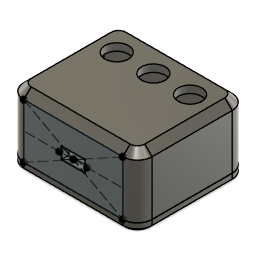
Button game box v5 (Autodesk Fusion 360 design; units mm, degrees)
Autodesk Fusion 360 part; units mm, degrees
sketch "Sketch2" plane through (0, 0, 0) normal (0, 1, 0) x (1, 0, 0)
  line L0 (-40.8037, -70.8274) -> (-40.8037, -26.2061)
  line L1 (-40.3037, -48.0998) -> (36.1963, -48.0998) construction
  line L2 (36.1963, -48.0998) -> (36.1963, -70.0998) construction
  line L3 (36.1963, -70.0998) -> (-40.3037, -70.0998) construction
  line L4 (-40.3037, -70.0998) -> (-40.3037, -48.0998) construction
  line L5 (-37.3037, -23.6203) -> (32.6963, -23.6203) construction
  line L6 (32.6963, -23.6203) -> (32.6963, -73.6203) construction
  line L7 (32.6963, -73.6203) -> (-37.3037, -73.6203) construction
  line L8 (-37.3037, -73.6203) -> (-37.3037, -23.6203) construction
  line L9 (36.1963, -48.0998) -> (-40.3037, -70.0998) construction
  line L10 (36.1963, -70.0998) -> (-40.3037, -48.0998) construction
  circle A0 centre (-2.0537, -59.0998) radius 2
  line L11 (30.6963, -23.6203) -> (30.6963, -73.6203) construction
  circle A1 centre (27.6642, -69.1203) radius 1.25
  line L12 (32.6963, -48.6203) -> (-37.3037, -48.6203) construction
  circle A2 centre (27.6642, -28.1203) radius 1.25
  line L13 (31.6963, -85.8274) -> (-35.8037, -85.8274)
  line L14 (-45.8037, -75.8274) -> (-45.8037, -21.2061)
  line L15 (-35.8037, -11.2061) -> (31.6963, -11.2061)
  line L16 (41.6963, -21.2061) -> (41.6963, -75.8274)
  arc A3 (-35.8037, -11.2061) -> (-45.8037, -21.2061) centre (-35.8037, -21.2061) ccw
  arc A4 (-45.8037, -75.8274) -> (-35.8037, -85.8274) centre (-35.8037, -75.8274) ccw
  arc A5 (31.6963, -85.8274) -> (41.6963, -75.8274) centre (31.6963, -75.8274) ccw
  arc A6 (41.6963, -21.2061) -> (31.6963, -11.2061) centre (31.6963, -21.2061) ccw
  line L17 (25.6941, -69.8252) -> (38.7674, -82.8985) construction
  line L18 (-35.8037, -75.8274) -> (-42.8747, -82.8985) construction
  line L19 (-35.8037, -75.8274) -> (-29.9973, -70.021) construction
  circle A7 centre (-39.3392, -79.3629) radius 2
  line L20 (25.6941, -69.8252) -> (15.45, -59.5811) construction
  circle A8 centre (35.2319, -79.3629) radius 2
  line L21 (38.7674, -14.135) -> (39.7345, -13.168) construction
  line L22 (39.7345, -13.168) -> (31.6963, -21.2061) construction
  circle A9 centre (35.2319, -17.6705) radius 2
  line L23 (-42.8747, -14.135) -> (-49.8297, -7.18) construction
  line L24 (-49.8297, -7.18) -> (-35.8037, -21.2061) construction
  circle A10 centre (-39.3392, -17.6705) radius 2
  line L25 (26.6963, -80.8274) -> (36.6963, -70.8274)
  line L26 (36.6963, -26.2061) -> (36.6963, -70.8274)
  line L27 (-40.8037, -70.8274) -> (-30.8037, -80.8274)
  line L28 (-40.8037, -26.2061) -> (-30.8037, -16.2061)
  line L29 (26.6963, -16.2061) -> (36.6963, -26.2061)
  line L30 (-30.8037, -16.2061) -> (26.6963, -16.2061)
  line L31 (26.6963, -80.8274) -> (-30.8037, -80.8274)
  circle A11 centre (-39.3392, -79.3629) radius 1.6
  circle A12 centre (-39.3392, -17.6705) radius 1.6
  circle A13 centre (35.2319, -17.6705) radius 1.6
  circle A14 centre (35.2319, -79.3629) radius 1.6
  dimension "d25" = 76.5
  dimension "d26" = 22
  dimension "d27" = 50
  dimension "d28" = 70
  dimension "d29" = 0.5
  dimension "d30" = 0.5
  dimension "d32" = 4
  dimension "d33" = 2.5
  dimension "d34" = 41
  dimension "d35" = 6
  dimension "d36" = 4
  dimension "d40" = 10
  dimension "d50" = 4
  dimension "d51" = 5
  dimension "d53" = 4
  dimension "d54" = 5
  dimension "d55" = 4
  dimension "d56" = 4
  dimension "d57" = 5
  dimension "d58" = 5
  dimension "d59" = 45
  dimension "d60" = 5
  dimension "d65" = 45
  dimension "d66" = 5
  dimension "d69" = 5
  dimension "d70" = 5
  dimension "d71" = 5
  dimension "d72" = 0.5
  dimension "d73" = 135
  dimension "d74" = 135
  dimension "d78" = 1
  dimension "d91" = 15.7276
  dimension "d105" = 3.2
  dimension "d106" = 3.2
  dimension "d107" = 3.2
  dimension "d108" = 3.2
  constraint vertical L26
  constraint horizontal L31
  constraint vertical L0
  constraint horizontal L1
  constraint vertical L2
  constraint horizontal L3
  constraint vertical L4
  constraint horizontal L5
  constraint vertical L6
  constraint horizontal L7
  constraint vertical L8
  constraint midpoint L9 A0.centre
  constraint coincident L5 L11.start
  constraint coincident L7 L11.end
  constraint perpendicular L7 L11
  constraint midpoint L6 L12.start
  constraint midpoint L8 L12.end
  constraint symmetric A1 L12 A2
  constraint tangent L15 A3
  constraint tangent L14 A3
  constraint tangent L14 A4
  constraint tangent L13 A4
  constraint equal A3 A4
  constraint tangent L13 A5
  constraint tangent L16 A5
  constraint equal A3 A5
  constraint tangent L16 A6
  constraint tangent L15 A6
  constraint equal A3 A6
  constraint midpoint A5 L17.end
  constraint midpoint A4 L18.end
  constraint parallel L18 L19
  constraint coincident L19 A7.centre
  constraint collinear L17 L20
  constraint coincident L20 A8.centre
  constraint midpoint A6 L21.start
  constraint coincident A6.centre L22.end
  constraint coincident L22 A9.centre
  constraint midpoint A3 L23.start
  constraint coincident A3.centre L24.end
  constraint coincident L23 A10.centre
  constraint horizontal L15
  constraint horizontal L30
  constraint midpoint A4.centre L27
  constraint perpendicular L17 L25
  constraint perpendicular L22 L29
  constraint perpendicular L24 L28
  constraint concentric A7 A11
  constraint concentric A10 A12
  constraint concentric A9 A13
  constraint concentric A8 A14
  measures "d25" distance of L2 L4
  measures "d26" distance of L1 L3
  measures "d27" distance of L5 L7
  measures "d28" distance of L6 L8
  measures "d29" distance of L2 L26
  measures "d30" distance of L0 L4
  measures "d32" diameter of A0
  measures "d33" diameter of A1
  measures "d34" distance of A1.centre A2.centre
  measures "d35" distance of L11 L26
  measures "d36" distance of L6 L26
  measures "d40" radius of A3
  measures "d50" diameter of A7
  measures "d51" distance of L18.end A7.centre
  measures "d53" diameter of A8
  measures "d54" distance of L17.end A8.centre
  measures "d55" diameter of A9
  measures "d56" diameter of A10
  measures "d57" distance of L23.start A10.centre
  measures "d58" distance of L21.start A9.centre
  measures "d59" angle of L25 L31
  measures "d60" distance of A8.centre L25
  measures "d65" angle of L27 L31
  measures "d66" distance of A7.centre L27
  measures "d69" distance of A10.centre L28
  measures "d70" distance of A9.centre L29
  measures "d71" distance of L15 L30
  measures "d72" distance of L7.end L27
  measures "d73" angle of L28 L30
  measures "d74" angle of L29 L30
  measures "d78" distance of L5.end L29
  measures "d91" distance of L3 L13
  measures "d105" diameter of A11
  measures "d106" diameter of A12
  measures "d107" diameter of A13
  measures "d108" diameter of A14
extrude "Extrude4" add sketch "Sketch2" against normal blind 5 contours L0 L25 L26 L27 L28 L29 L30 L31 | A0 | A1 | A2 | L13 L14 L15 L16 A3 A4 A5 A6 | A7 | A8 | A9 | A10 | A11 | A12 | A13 | A14 makes body 1
extrude "Extrude5" add sketch "Sketch2" against normal blind 37 from surface at -5 contours L13 L14 L15 L16 A3 A4 A5 A6 | A7 | A8 | A9 | A10 | A11 | A12 | A13 | A14 bodies 1
sketch "Sketch1" plane through (0, 0, 0) normal (0, 1, 0) x (1, 0, 0)
  arc A0 (31.6963, -85.8274) -> (41.6963, -75.8274) centre (31.6963, -75.8274) ccw
  line L0 (41.6963, -75.8274) -> (41.6963, -21.2061)
  arc A1 (41.6963, -21.2061) -> (31.6963, -11.2061) centre (31.6963, -21.2061) ccw
  line L1 (31.6963, -11.2061) -> (-35.8037, -11.2061)
  arc A2 (-35.8037, -11.2061) -> (-45.8037, -21.2061) centre (-35.8037, -21.2061) ccw
  line L2 (-45.8037, -21.2061) -> (-45.8037, -75.8274)
  arc A3 (-45.8037, -75.8274) -> (-35.8037, -85.8274) centre (-35.8037, -75.8274) ccw
  line L3 (-35.8037, -85.8274) -> (31.6963, -85.8274)
  circle A4 centre (22.9463, -31.2061) radius 8
  circle A5 centre (-2.0537, -31.2061) radius 8
  arc A6 (-35.0537, -31.2061) -> (-19.0537, -31.2061) centre (-27.0537, -31.2061) ccw
  arc A7 (-19.0537, -31.2061) -> (-35.0537, -31.2061) centre (-27.0537, -31.2061) ccw
  line L4 (-19.0537, -31.2061) -> (-45.8037, -31.2061) construction
  line L5 (-10.0537, -31.2061) -> (-19.0537, -31.2061) construction
  line L6 (41.6963, -31.2061) -> (14.9463, -31.2061) construction
  line L7 (5.9463, -31.2061) -> (-10.0537, -31.2061) construction
  line L8 (14.9463, -31.2061) -> (5.9463, -31.2061) construction
  line L9 (-2.0537, -85.8274) -> (-2.0537, -11.2061) construction
  point P0 (-2.0537, -48.5167)
  dimension "d79" = 16
  dimension "d80" = 16
  dimension "d81" = 16
  dimension "d82" = 20
  dimension "d83" = 25
  constraint coincident L0 L6.start
  constraint coincident L2 L4.end
  constraint perpendicular L2 L6
  constraint coincident A4.centre L6
  constraint coincident A5.centre L6
  constraint coincident A6.centre L6
  constraint coincident A6.end L6
  constraint coincident A6.start L6
  constraint concentric A6 A7
  constraint coincident A5 L5.start
  constraint coincident A4 L6.end
  constraint coincident A5 L7.start
  constraint collinear L6 L8
  constraint collinear L7 L8
  constraint collinear L5 L7
  constraint collinear L4 L5
  constraint equal L5 L8
  constraint midpoint L3 L9.start
  constraint midpoint L1 L9.end
  constraint coincident A5.centre L9
  measures "d79" diameter of A4
  measures "d80" diameter of A5
  measures "d81" diameter of A6
  measures "d82" distance of L1 L5
  measures "d83" distance of A5.centre A6.centre
extrude "Extrude6" cut sketch "Sketch1" against normal up to surface (5 mm away) contours A4 | A5 | A6 A7 bodies 1
chamfer "Chamfer2" distance 5 angle 45 8 edges at (-2.0537, 0, 85.8274) (-42.8747, 0, 82.8985) (-45.8037, 0, 48.5167) (-42.8747, 0, 14.135) (-2.0537, 0, 11.2061) (38.7674, 0, 14.135) (41.6963, 0, 48.5167) (38.7674, 0, 82.8985) on bodies 1
extrude "Extrude7" cut sketch "Sketch2" along normal blind 13 from surface at -42 contours A7 | A8 | A9 | A10 | A11 | A12 | A13 | A14 bodies 1
extrude "Extrude9" cut sketch "Sketch2" along normal blind 3.5 from surface at -5 contours A0 bodies 1
extrude "Extrude8" add sketch "Sketch2" against normal blind 5 from surface at -42.1 separate body contours L0 L25 L26 L27 L28 L29 L30 L31 | A0 | A1 | A2 | L13 L14 L15 L16 A3 A4 A5 A6 | A7 | A8 | A9 | A10 makes body 2
extrude "Extrude10" cut sketch "Sketch2" against normal blind 3.5 from surface at -42.1 contours A1 | A2 bodies 2
chamfer "Chamfer3" distance 1.5 angle 45 8 edges at (41.6963, -47.1, 48.5167) (38.7674, -47.1, 82.8985) (-2.0537, -47.1, 85.8274) (-42.8747, -47.1, 82.8985) (-45.8037, -47.1, 48.5167) (-42.8747, -47.1, 14.135) (-2.0537, -47.1, 11.2061) (38.7674, -47.1, 14.135) on bodies 2
chamfer "Chamfer3" distance 1 angle 45 4 edges at (-40.8309, -47.1, 18.2491) (-40.8309, -47.1, 79.9415) (33.7401, -47.1, 79.9415) (33.7401, -47.1, 18.2491) on bodies 2
sketch "Sketch3" plane through (0, 0, 85.8274) normal (0, 0, 1) x (1, 0, 0)
  line L0 (31.6963, -5) -> (-35.8037, -5)
  line L1 (-35.8037, -5) -> (-35.8037, -42)
  line L2 (-35.8037, -42) -> (31.6963, -42)
  line L3 (31.6963, -42) -> (31.6963, -5)
  line L4 (31.6963, -5) -> (-35.8037, -42) construction
  line L5 (-35.8037, -5) -> (31.6963, -42) construction
  line L6 (5.9463, -19.5) -> (-10.0537, -19.5)
  line L7 (-10.0537, -19.5) -> (-10.0537, -27.5)
  line L8 (-10.0537, -27.5) -> (5.9463, -27.5)
  line L9 (5.9463, -27.5) -> (5.9463, -19.5)
  line L10 (5.9463, -19.5) -> (-10.0537, -27.5) construction
  line L11 (-10.0537, -19.5) -> (5.9463, -27.5) construction
  line L12 (-2.0537, -23.5) -> (31.6963, -23.5) construction
  line L13 (-2.0537, -23.5) -> (-35.8037, -23.5) construction
  circle A0 centre (7.4463, -23.5) radius 0.8
  circle A1 centre (-11.5537, -23.5) radius 0.8
  point P0 (-2.0537, -23.5)
  dimension "d92" = 16
  dimension "d93" = 8
  dimension "d94" = 9.5
  dimension "d95" = 9.5
  dimension "d96" = 1.6
  dimension "d97" = 1.6
  constraint coincident L0.start L3.end
  constraint coincident L1.end L2.start
  constraint coincident L0.end L1.start
  constraint coincident L2.end L3.start
  constraint horizontal L6
  constraint perpendicular L6 L7
  constraint parallel L6 L8
  constraint parallel L7 L9
  constraint coincident L10 P0
  constraint coincident L11 P0
  constraint midpoint L5 P0
  constraint coincident P0 L12.start
  constraint midpoint L3 L12.end
  constraint midpoint L1 L13.end
  constraint coincident L12 A0.centre
  constraint coincident L13 A1.centre
  measures "d92" distance of L7 L9
  measures "d93" distance of L6 L8
  measures "d94" distance of P0 A0.centre
  measures "d95" distance of P0 A1.centre
  measures "d96" diameter of A0
  measures "d97" diameter of A1
extrude "Extrude11" cut sketch "Sketch3" against normal up to surface (5 mm away) contours L6 L7 L8 L9 bodies 1
extrude "Extrude12" cut sketch "Sketch3" against normal blind 4 contours A0 | A1 bodies 1
equation "buttonHoleD = 16 mm"
equation "wallThickness = 5 mm"
equation "d32 = threadedInsertHoleD"
equation "d50 = threadedInsertHoleD"
equation "d51 = threadedInsertHoleD / 2 + threadedInsertWall"
equation "threadedInsertHoleD = 4 mm"
equation "d53 = threadedInsertHoleD"
equation "d54 = threadedInsertHoleD / 2 + threadedInsertWall"
equation "d55 = threadedInsertHoleD"
equation "d56 = threadedInsertHoleD"
equation "d57 = threadedInsertHoleD / 2 + threadedInsertWall"
equation "d58 = threadedInsertHoleD / 2 + threadedInsertWall"
equation "d60 = threadedInsertHoleD / 2 + threadedInsertWall"
equation "threadedInsertWall = 3 mm"
equation "d66 = threadedInsertHoleD / 2 + threadedInsertWall"
equation "d69 = threadedInsertHoleD / 2 + threadedInsertWall"
equation "d70 = threadedInsertHoleD / 2 + threadedInsertWall"
equation "d71 = wallThickness"
equation "d76 = -wallThickness"
equation "d79 = buttonHoleD"
equation "d80 = buttonHoleD"
equation "d81 = buttonHoleD"
equation "d82 = 15 mm + wallThickness"
equation "d100 = -wallThickness + 1 mm"
equation "screwClearanceHoleD = 3.2 mm"
equation "d105 = screwClearanceHoleD"
equation "d106 = screwClearanceHoleD"
equation "d107 = screwClearanceHoleD"
equation "d108 = screwClearanceHoleD"
named bodies: "Main body", "Cover"
